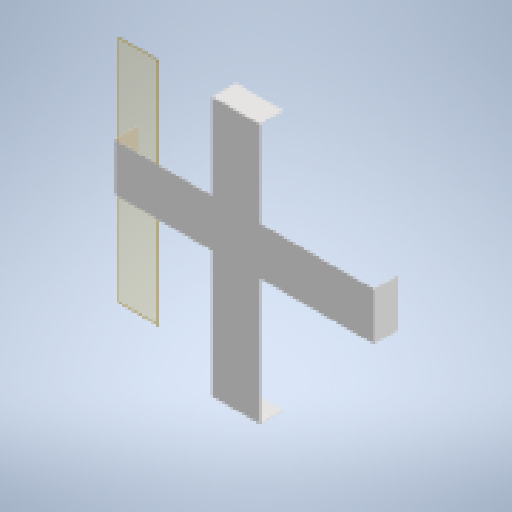
# Autodesk Inventor part: Brush_holder
Saved by Autodesk Inventor 2024 (Build 280153000, 153)
## iProperties
Created: 2024-04-11
Part Number: Brush_holder
Material: Generic
Document SubType Name: Sheet Metal
Designer: teeta
Density: 1 g/cm^3
Sheet Metal Rule: Default_mm
Appearance: Default
Author: teeta
Autodesk Inventor part; units mm, degrees
ref_plane "YZ Plane" through (0, 0, 0) normal (1, 0, 0) x (0, 1, 0)
ref_plane "XZ Plane" through (0, 0, 0) normal (0, 1, 0) x (-1, 0, 0)
ref_plane "XY Plane" through (0, 0, 0) normal (0, 0, 1) x (1, 0, 0)
ref_plane "Work Plane1" through (0, 0, 0) normal (0, 0, 1) x (1, 0, 0)
sketch "Sketch1" plane through (0, 0, 0) normal (0, 0, 1) x (1, 0, 0)
  line L0 (230.575, 85.4) -> (230.575, 135.4)
  line L1 (-46.45, 135.4) -> (-46.45, 85.4)
  line L2 (58.575, -49.625) -> (108.575, -49.625)
  line L3 (108.575, 227.4) -> (58.575, 227.4)
  line L4 (-622.225, -47.625) -> (228.575, -47.625)
  line L5 (-44.45, 0) -> (-44.45, 225.4)
  line L6 (180.95, 225.4) -> (-44.45, 225.4)
  line L7 (228.575, -47.625) -> (228.575, 1203.175)
  line L8 (-46.45, 85.4) -> (58.575, 85.4)
  line L9 (108.575, 85.4) -> (230.575, 85.4)
  line L10 (108.575, -49.625) -> (108.575, 85.4)
  line L11 (108.575, 135.4) -> (108.575, 227.4)
  line L12 (58.575, 227.4) -> (58.575, 135.4)
  line L13 (58.575, 85.4) -> (58.575, -49.625)
  line L14 (230.575, 135.4) -> (108.575, 135.4)
  line L15 (58.575, 135.4) -> (-46.45, 135.4)
  point P0 (0, 0)
  point P1 (83.575, 227.4)
  point P2 (83.575, -49.625)
  dimension "d16" = 2
  dimension "d17" = 2
  dimension "d18" = 2
  dimension "d19" = 2
  dimension "d20" = 92
  dimension "d21" = 122
  dimension "d22" = 105.025
  dimension "d23" = 135.025
  dimension "d24" = 50
  dimension "d25" = 50
  dimension "d26" = 50
  measures "d16" distance from line of L4 point (83.575, -49.625)
  measures "d17" distance between parallel lines of L5 L1
  measures "d18" distance between parallel lines of L6 L3
  measures "d19" distance between parallel lines of L7 L0
  measures "d20" distance of L11.start L3.start
  measures "d21" distance of L9.start L0.start
  measures "d22" distance of L12.end L1.start
  measures "d23" distance of L8.end L2.start
  measures "d24" distance of L1.start L1.end
  measures "d25" distance of L2.start L2.end
  measures "d26" distance of L3.start L3.end
extrude "Plate1" add sketch "Sketch1" along normal blind 0.5 contours L9 L7 L14 L0 | L9 L10 L4 L13 L8 L5 L15 L12 L6 L11 L14 L7 | L10 L2 L13 L4 | L6 L12 L3 L11 | L8 L1 L15 L5
sketch "Sketch3" plane through (108.575, -49.125, 0.5) normal (0, -1, 0) x (1, 0, 0)
  line L0 (-50, 0) -> (0, 0)
  line L1 (0, 0) -> (0, 25)
  line L2 (0, 25) -> (-50, 25)
  line L3 (-50, 25) -> (-50, 0)
  constraints: 6 end point, 1 horizontal, 1 perpendicular, 1 vertical
edge flange "Flange2" height 25 angle 90 thickness 0.5 bend radius 0.5 thickness toward (0, -1, 0) relief tear relief width 0.5 relief depth 0.25 corner gap 0.5 corner form 0 edges at (83.575, -49.625, 0.5) (230.575, 110.4, 0.5) (83.575, 227.4, 0.5) (-46.45, 110.4, 0.5) wall of the first edge with corners at (58.575, -49.125, 0.5) (108.575, -49.125, 0.5) (108.575, -49.125, -24.5) (58.575, -49.125, -24.5)
bend "Bend2"
corner "Corner2"
equation "\"d4\" = Thickness"
equation "\"d27\" = BendReliefWidth"
equation "\"d28\" = BendReliefDepth"
equation "\"d29\" = MinimumRemnant"
equation "\"d30\" = TransitionRadius"
equation "\"d33\" = BendRadius"
equation "\"d34\" = CornerReliefSize"
equation "\"d35\" = GapSize"
equation "\"d36\" = JacobiRadiusSize"
equation "\"BendRadius\" = Thickness"
equation "\"BendReliefWidth\" = Thickness"
equation "\"BendReliefDepth\" = 0.5 * Thickness"
equation "\"CornerReliefSize\" = 4 * Thickness"
equation "\"MinimumRemnant\" = 2 * Thickness"
equation "\"TransitionRadius\" = BendRadius"
equation "\"JacobiRadiusSize\" = BendRadius"
equation "\"GapSize\" = Thickness"
equation "\"Thickness\" = 0.5"
body "Solid1"
